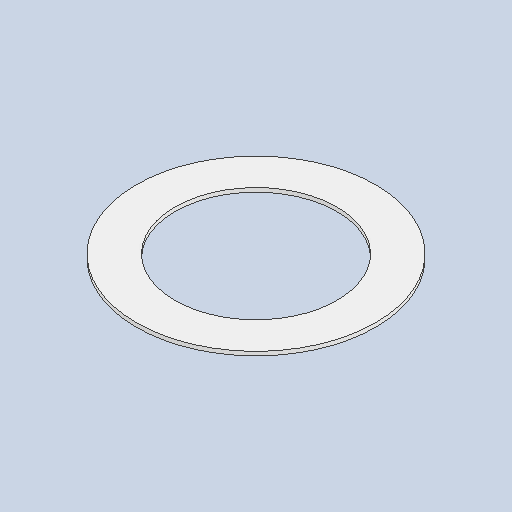
# Autodesk Inventor part: 2030 Teflon Sheet
Saved by Autodesk Inventor 2026.1 (Build 301233000, 233)
## iProperties
Created: 2023-10-27
Part Number: 2030 Teflon Sheet
Material: ABS Plastic
Document SubType Name: Modeling
Designer: chanh
Density: 1.06 g/cm^3
Appearance: White
Author: chanh
Autodesk Inventor part; units mm, degrees
ref_plane "YZ Plane" through (0, 0, 0) normal (1, 0, 0) x (0, 1, 0)
ref_plane "XZ Plane" through (0, 0, 0) normal (0, 1, 0) x (-1, 0, 0)
ref_plane "XY Plane" through (0, 0, 0) normal (0, 0, 1) x (1, 0, 0)
sketch "Sketch1" plane through (0, 0, 0) normal (0, 1, 0) x (-1, 0, 0)
  circle A0 centre (0, 0) radius 15
  circle A1 centre (0, 0) radius 10.16
  dimension "d0" = 30
  dimension "d1" = 20.32
  constraints: 2 centre point, 2 coincident
  measures "d0" diameter of A0
  measures "d1" diameter of A1
extrude "Extrusion1" add sketch "Sketch1" along normal blind 0.5
body "Solid1"
